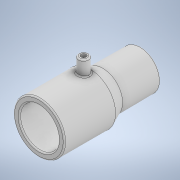
# Autodesk Inventor part: puntopresion2
Saved by Autodesk Inventor 2020.2 (Build 242310000, 310)
## iProperties
Created: 2020-08-02
Part Number: puntopresion2
Material: Generic
Document SubType Name: Modeling
Designer: JK
Density: 1 g/cm^3
Appearance: Default
Author: JK
Autodesk Inventor part; units mm, degrees
ref_plane "YZ Plane" through (0, 0, 0) normal (1, 0, 0) x (0, 1, 0)
ref_plane "XZ Plane" through (0, 0, 0) normal (0, 1, 0) x (-1, 0, 0)
ref_plane "XY Plane" through (0, 0, 0) normal (0, 0, 1) x (1, 0, 0)
sketch "Sketch7" plane through (0, 0, 0) normal (1, 0, 0) x (0, 1, 0)
  line L0 (0, 81.0588) -> (10, 81.0588)
  line L1 (10, 81.0588) -> (10, 66.0588)
  line L2 (7.6, 81.0588) -> (7.75, 66.0588)
  line L3 (0, 0) -> (0, 99.048)
  line L4 (10, 66.0588) -> (10, 61.0588)
  line L5 (7.75, 66.0588) -> (7.75, 61.0588)
  line L6 (10, 61.0588) -> (7.75, 56.0588)
  line L7 (7.75, 61.0588) -> (5.5, 56.0588)
  line L8 (7.75, 56.0588) -> (7.6, 41.0588)
  line L9 (5.5, 56.0588) -> (5.5, 41.0588)
  line L10 (5.5, 41.0588) -> (7.6, 41.0588)
  dimension "d12" = 10
  dimension "d13" = 15
  dimension "d14" = 7.6
  dimension "d15" = 7.75
  dimension "d16" = 5
  dimension "d18" = 7.75
  dimension "d19" = 5.5
  dimension "d20" = 5
  dimension "d21" = 15
  dimension "d22" = 7.6
  constraints: 22 end point, 5 vertical, 3 horizontal alignment, 2 horizontal, 1 point on line, 1 vertical alignment
  measures "d12" distance of L0.start L0.end
  measures "d13" distance of L1.end L0.end
  measures "d14" distance from line of L3 L2.start
  measures "d15" distance from line of L3 L2.end
  measures "d16" distance of L4.end L1.end
  measures "d18" distance from line of L3 L6.end
  measures "d19" distance from line of L3 L7.end
  measures "d20" vertical distance of L4.end L6.end
  measures "d21" distance of L9.end L7.end
  measures "d22" distance from line of L3 L8.end
revolve "Revolution1" add sketch "Sketch7" angle 360 about axis through (0, 0, 0) along (0, 0, 1)
sketch "Sketch8" plane through (0, 0, 0) normal (0, 1, 0) x (-1, 0, 0)
  circle A0 centre (0, 63.5588) radius 2
  line L0 (-10, 61.0588) -> (10, 61.0588) projected
  point P0 (0, 0)
  dimension "d24" = 4
  dimension "d25" = 2.5
  constraints: 1 centre point
  measures "d24" diameter of A0
  measures "d25" distance from line of L0 A0.centre
extrude "Extrusion4" add sketch "Sketch8" along normal blind 15.75
sketch "Sketch9" plane through (0, 15.75, 63.5588) normal (0, 1, 0) x (1, 0, 0)
  circle A0 centre (0, 0) radius 1
  point P0 (0, 63.5588)
  dimension "d28" = 2
  constraints: 1 centre point
  measures "d28" diameter of A0
extrude "Extrusion5" cut sketch "Sketch9" against normal blind 13
sketch "Sketch11" plane through (0, 0, 0) normal (1, 0, 0) x (0, 1, 0)
  line L0 (7.75, 61.0588) -> (7.75, 66.0588) projected
  line L1 (0, 61.5588) -> (0, 65.5588) projected
  line L2 (7.75, 61.0588) -> (0, 61.0588)
  line L3 (0, 61.0588) -> (0, 65.5588)
  line L4 (0, 65.5588) -> (7.75, 65.5588)
  line L5 (7.75, 65.5588) -> (7.75, 61.0588)
  line L6 (-7.75, 66.0588) -> (7.75, 66.0588) projected
  line L7 (-10, 61.0588) -> (10, 61.0588) projected
  line L8 (7.75, 66.0588) -> (7.25, 66.0588)
  line L9 (7.25, 66.0588) -> (7.25, 61.0588)
  line L10 (7.25, 61.0588) -> (7.75, 61.0588)
  line L11 (7.75, 61.0588) -> (7.75, 66.0588)
  point P0 (0, 0)
  point P1 (7.25, 65.5588)
  dimension "d35" = 0.5
  constraints: 16 end point, 4 parallel, 2 horizontal, 2 perpendicular, 2 point on line
  measures "d35" distance between parallel lines of L0 L9
revolve "Revolution2" cut sketch "Sketch11" angle 360 about axis through (0, 0, 61.0588) along (0, 0, 1) contours L2 L3 L1 L4 L9
fillet "Fillet2" radius 0.5 8 edges at (0, -7.6, 81.0588) (0, -10, 81.0588) (2, 15.75, 63.5588) (-1.5156, 9.8845, 64.8638) (-1.5148, 9.8846, 62.2529) (2, 9.798, 63.559) (0, -5.5, 41.0588) (0, -7.6, 41.0588)
body "Solid2"
